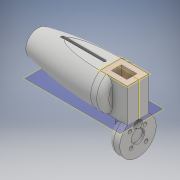
# Autodesk Inventor part: Halterung Motor Neu
Saved by Autodesk Inventor 2019 (Build 230136000, 136)
## iProperties
Created: 2017-06-08
Part Number: Halterung Motor Neu
Material: Allgemein
Document SubType Name: Modeling
Designer: eule-3
Density: 1 g/cm^3
Appearance: Vorgabe
Author: eule-3
Autodesk Inventor part; units mm, degrees
ref_plane "YZ Plane" through (0, 0, 0) normal (1, 0, 0) x (0, 1, 0)
ref_plane "XZ Plane" through (0, 0, 0) normal (0, 1, 0) x (-1, 0, 0)
ref_plane "XY Plane" through (0, 0, 0) normal (0, 0, 1) x (1, 0, 0)
sketch "Skizze1" plane through (0, 0, 0) normal (0, 0, 1) x (1, 0, 0)
  point P0 (0, 0)
sketch "Skizze2" plane through (0, 0, 0) normal (0, 0, 1) x (1, 0, 0)
  line L0 (0, 0) -> (22.5, 0)
  line L1 (22.5, 0) -> (22.5, 17.5)
  line L2 (22.5, 17.5) -> (0, 17.5)
  line L3 (0, 17.5) -> (0, 0)
  dimension "d0" = 17.5
  dimension "d1" = 22.5
  constraints: 8 end point, 2 parallel, 1 horizontal, 1 perpendicular
  measures "d0" distance of L0.end L1.end
  measures "d1" distance of L1.end L2.end
extrude "Extrusion1" add sketch "Skizze2" along normal blind 28
sketch "Skizze3" plane through (0, 17.5, 0) normal (0, 1, 0) x (1, 0, 0)
  point P0 (0, 0)
sketch "Skizze4" plane through (22.5, 0, 0) normal (1, 0, 0) x (0, 0, -1)
  circle A0 centre (12.1835, 8.75) radius 15
  line L0 (0, 17.5) -> (-28, 17.5) projected
  line L1 (0, 0) -> (-28, 0) projected
  dimension "d4" = 30
  dimension "d5" = 8.75
  dimension "d6" = 8.75
  dimension "d7" = 15
  constraints: 1 centre point
  measures "d4" diameter of A0
  measures "d5" distance from line of A0.centre L0
  measures "d6" distance from line of A0.centre L1
  measures "d7" distance of A0.centre L0.start
extrude "Extrusion2" cut sketch "Skizze4" against normal blind 22.5
sketch "Skizze5" plane through (22.5, 0, 28) normal (1, 0, 0) x (0, 0, -1)
  circle A0 centre (40.1835, 8.75) radius 15
  line L0 (28, 17.5) -> (0, 17.5) projected
  point P0 (28, 0)
  dimension "d10" = 30
  dimension "d11" = 8.75
  dimension "d12" = 15
  constraints: 1 centre point
  measures "d10" diameter of A0
  measures "d11" distance from line of L0 A0.centre
  measures "d12" distance of L0.start A0.centre
extrude "Extrusion3" add sketch "Skizze5" against normal blind 22.5
sketch "Skizze6" plane through (22.5, 0, 28) normal (1, 0, 0) x (0, 0, -1)
  point P0 (28, 0)
sketch "Skizze7" plane through (0, 0, 28) normal (-1, 0, 0) x (0, 0, 1)
  circle A0 centre (-40.1835, 8.75) radius 15
  line L0 (-28, 0) -> (0, 0) projected
  dimension "d15" = 30
  dimension "d16" = 8.75
  dimension "d17" = 15
  constraints: 1 centre point
  measures "d15" diameter of A0
  measures "d16" distance from line of L0 A0.centre
  measures "d17" distance of A0.centre L0.start
extrude "Extrusion4" cut sketch "Skizze7" against normal blind 12.5
sketch "Skizze8" plane through (0, 0, 28) normal (-1, 0, 0) x (0, 0, 1)
  line L0 (-28, 17.4854) -> (-24, 17.4854)
  line L1 (-24, 17.4854) -> (-24, 0)
  line L2 (-24, 0) -> (-28, 0)
  line L3 (-28, 0) -> (-28, 17.4854)
  constraints: 8 end point, 2 parallel, 1 horizontal, 1 perpendicular
extrude "Extrusion5" add sketch "Skizze8" against normal blind 12.5
sketch "Skizze9" plane through (12.5, 0, 28) normal (-1, 0, 0) x (0, 0, 1)
  point P0 (-28, 0)
sketch "Skizze10" plane through (12.5, 0, 28) normal (-1, 0, 0) x (0, 0, 1)
  line L0 (-28, 17.5) -> (0, 17.5) projected
  arc A0 (-28, 17.5) -> (-28, 0) centre (-40.1835, 8.75) ccw projected
  line L1 (-28, 0) -> (-28, 17.4854) projected
  line L2 (-40.1835, 8.75) -> (-28, 8.7427)
  line L3 (-40.1835, 23.75) -> (-40.1835, 8.75)
  line L4 (-55.1835, 8.75) -> (-40.1835, 8.75)
  line L5 (-40.1835, 8.75) -> (-40.1835, -6.25)
  point P0 (-34.5249, 14.4052)
  point P1 (-33.468, 2.0305)
  point P2 (-46.901, 15.4675)
  point P3 (-45.8403, 3.0931)
  dimension "d38" = 9.5
  constraints: 8 end point, 3 point on circle, 1 horizontal, 1 midpoint, 1 perpendicular, 1 point on line, 1 vertical
  measures "d38" distance of L2.start point (-46.901, 15.468)
hole "Bohrung1" at (12.5, 15.4675, -18.901) at (12.5, 2.0305, -5.468) at (12.5, 3.0931, -17.8403) at (12.5, 14.4052, -6.5249) direction (1, 0, 0) diameter 3 end through all
sketch "Skizze11" plane through (12.5, 0, 28) normal (-1, 0, 0) x (0, 0, 1)
  point P0 (-28, 0)
sketch "Skizze12" plane through (0, 0, 28) normal (0, 0, 1) x (1, 0, 0)
  line L0 (4.8, 12.85) -> (17.5, 12.85)
  line L1 (17.5, 12.85) -> (17.5, 4.65)
  line L2 (17.5, 4.65) -> (4.8, 4.65)
  line L3 (4.8, 4.65) -> (4.8, 12.85)
  line L4 (22.5, 17.5) -> (0, 17.5) projected
  line L5 (22.5, 0) -> (22.5, 17.5) projected
  line L6 (0, 17.5) -> (0, 0) projected
  line L7 (0, 0) -> (22.5, 0) projected
  dimension "d78" = 4.65
  dimension "d79" = 4.65
  dimension "d111" = 5
  dimension "d112" = 12.7
  constraints: 8 end point, 2 parallel, 1 horizontal, 1 perpendicular
  measures "d78" distance between parallel lines of L4 L0
  measures "d79" distance between parallel lines of L7 L2
  measures "d111" distance between parallel lines of L5 L1
  measures "d112" distance of L1.end L2.end
extrude "Extrusion6" cut sketch "Skizze12" against normal blind 30 contours L0 L1 L2 L3
sketch "Skizze13" plane through (12.5, 0, 28) normal (-1, 0, 0) x (0, 0, 1)
  circle A0 centre (-31.75, 8.75) radius 2.25
  line L0 (-30, 12.85) -> (-30, 4.65) projected
  point P0 (-28, 0)
  dimension "d71" = 1.75
  constraints: 1 centre point, 1 coincident
  measures "d71" distance from line of L0 A0.centre
extrude "Extrusion7" cut sketch "Skizze13" against normal blind 10
sketch "Skizze14" plane through (22.5, 0, 28) normal (1, 0, 0) x (0, 0, -1)
  line L0 (28, 17.5) -> (0, 17.5) projected
  circle A0 centre (31.75, 8.75) radius 2.25 projected
  arc A1 (28, 0) -> (28, 17.5) centre (40.1835, 8.75) ccw projected
  circle A2 centre (40.1835, 8.75) radius 5
  dimension "d57" = 10
  constraints: 1 centre point, 1 coincident
  measures "d57" diameter of A2
extrude "Extrusion8" cut sketch "Skizze14" against normal blind 1.5 contours A2
chamfer "Fase1" distance 0.5 angle 45 1 edges at (22.5, 8.75, -7.1835)
chamfer "Fase2" distance 0.5 angle 45 4 edges at (12.5, 15.4675, -20.401) (12.5, 14.4052, -8.0249) (12.5, 2.0305, -6.968) (12.5, 3.0931, -19.3403)
sketch "Skizze16" plane through (12.5, 0, 28) normal (-1, 0, 0) x (0, 0, 1)
  circle A0 centre (-31.75, 8.75) radius 2.25 projected
  line L0 (-30, 4.65) -> (-30, 7.3358) projected
  line L1 (-31.75, 10.825) -> (-30, 10.825)
  line L2 (-30, 10.825) -> (-30, 5.9929)
  line L3 (-30, 5.9929) -> (-31.75, 5.9929)
  line L4 (-31.75, 5.9929) -> (-31.75, 10.825)
  point P0 (-28, 0)
  point P1 (-31.75, 6.5)
  constraints: 8 end point, 2 parallel, 1 coincident, 1 horizontal, 1 midpoint, 1 perpendicular, 1 other
extrude "Extrusion9" cut sketch "Skizze16" against normal blind 5 contours L0 L3 L4 A0 | A0 L4 L1 L2 | A0 L1 L2
sketch "Skizze17" plane through (0, 0, 28) normal (0, 0, 1) x (1, 0, 0)
  point P0 (0, 0)
sketch "Skizze18" plane through (0, 0, -2) normal (0, 0, 1) x (1, 0, 0)
  line L0 (12.5, 6.5) -> (17.5, 6.5) projected
  line L1 (12.5, 5.9929) -> (17.5, 5.9929) projected
  line L2 (12.5, 6.5) -> (17.5, 6.5)
  line L3 (17.5, 6.5) -> (17.5, 5.9929)
  line L4 (17.5, 5.9929) -> (12.5, 5.9929)
  line L5 (12.5, 5.9929) -> (12.5, 6.5)
  point P0 (0, 0)
  constraints: 8 end point, 2 parallel, 1 horizontal, 1 perpendicular
extrude "Extrusion10" add sketch "Skizze18" against normal blind 5
sketch "Skizze19" plane through (22.5, 0, 28) normal (1, 0, 0) x (0, 0, -1)
  circle A0 centre (31.7095, 8.8101) radius 3.5
  point P0 (28, 0)
  dimension "d80" = 7
  constraints: 1 centre point
  measures "d80" diameter of A0
extrude "Extrusion11" cut sketch "Skizze19" against normal blind 5
sketch "Skizze20" plane through (0, 0, 28) normal (0, 0, 1) x (1, 0, 0)
  line L0 (17.5, 4.65) -> (4.8, 4.65) projected
  line L1 (4.8, 12.85) -> (17.5, 12.85) projected
  line L2 (4.8, 4.65) -> (4.8, 12.85) projected
  line L3 (17.5, 12.85) -> (17.5, 4.65) projected
  point P0 (0, 0)
sketch "Skizze21" plane through (0, 0, 28) normal (-1, 0, 0) x (0, 0, 1)
  line L0 (-28, 0) -> (-28, 17.4854) projected
  line L1 (-28, 17.5) -> (0, 17.5) projected
  line L2 (-28, 0) -> (0, 0)
  line L3 (0, 0) -> (0, 17.5)
  line L4 (0, 17.5) -> (-28, 17.5)
  line L5 (-28, 17.5) -> (-28, 0)
  arc A0 (0, 17.5) -> (-28, 17.5) centre (-14, 8.75) ccw
  arc A1 (-28, 0) -> (0, 0) centre (-14, 8.75) ccw
  point P0 (-28.6212, 17.5)
  dimension "d85" = 28
  dimension "d86" = 17.5
  dimension "d87" = 16.5095
  constraints: 8 end point, 4 point on circle, 2 centre point, 2 coincident, 2 parallel, 1 horizontal, 1 perpendicular
  measures "d85" distance between parallel lines of L3 L0
  measures "d86" distance between parallel lines of L2 L1
  measures "d87" radius of A0
extrude "Extrusion12" add sketch "Skizze21" against normal blind 10 contours L2 A1 | A0 L1
fillet "Rundung1" radius 5 2 edges at (10, -7.7595, 14) (10, 25.2595, 14)
sketch "Skizze22" plane through (0, 0, 28) normal (0, 0, 1) x (1, 0, 0)
  point P0 (0, 0)
ref_plane "Arbeitsebene1" through (13, 8.75, 0) normal (0, -1, 0) x (1, 0, 0)
sketch "Skizze23" plane through (13, 8.75, 0) normal (0, -1, 0) x (1, 0, 0)
  line L0 (-13, 28) -> (-13, 0) projected
  line L1 (-73, 14) -> (-73, 24)
  line L2 (-13, 14) -> (-13, 30.5095)
  line L3 (-13, 0) -> (-8, 0) projected
  arc A0 (-13, 30.5095) -> (-73, 24) centre (-13, -249.2642) ccw
  line L4 (-73, 14) -> (-13, 14)
  dimension "d92" = 60
  dimension "d93" = 10
  dimension "d94" = 16.5095
  dimension "d95" = 14
  constraints: 6 end point, 2 point on circle, 2 vertical, 1 centre point, 1 line through centre, 1 midpoint
  measures "d92" distance of L2.start L1.start
  measures "d93" distance of L1.start L1.end
  measures "d94" distance of L2.start L2.end
  measures "d95" distance from line of L3 L1.start
revolve "Umdrehung1" add sketch "Skizze23" angle 360 about axis through (-60, 8.75, 14) along (1, 0, 0) separate body
sketch "Skizze25" plane through (0, 8.75, 14) normal (1, 0, 0) x (0, 0, -1)
  point P0 (14, -8.75)
ref_plane "Arbeitsebene2" through (0, 0, 28) normal (0, 0, 1) x (1, 0, 0)
ref_plane "Arbeitsebene3" through (6.25, 17.4854, 0) normal (0, 0, -1) x (-1, 0, 0)
split "Trennen3" plane through (6.25, 17.4854, 0) removes the side toward (0, 0, -1) bodies 2
split "Trennen4" plane through (0, 0, 28) removes the side toward (0, 0, 1) bodies 2
sketch "Skizze27" plane through (-60, 8.75, 14) normal (-1, 0, 0) x (0, 0, 1)
  line L0 (14, 4.1) -> (-14, 4.1) projected
  line L1 (-14, -8.7501) -> (-14, 8.7501) projected
  point P0 (-14, -8.75)
  point P1 (0, 0)
  point P2 (0, 4.1)
  point P3 (-14, 0)
  constraints: 2 midpoint, 1 horizontal alignment, 1 vertical alignment
hole "Bohrung2" at (-60, 8.75, 14) direction (1, 0, 0) diameter 11 depth 50 tip angle 118 counterbore diameter 13 counterbore depth 8 bodies 2
sketch "Skizze28" plane through (0, -0.0001, 0) normal (0, 0, -1) x (-1, 0, 0)
  line L0 (5, 8.7501) -> (40, 8.7501) construction
  line L1 (5, 7.7501) -> (40, 7.7501)
  line L2 (40, 9.7501) -> (5, 9.7501)
  arc A0 (5, 9.7501) -> (5, 7.7501) centre (5, 8.7501) ccw
  arc A1 (40, 7.7501) -> (40, 9.7501) centre (40, 8.7501) ccw
  line L3 (76.5004, 8.7501) -> (-39.0025, 8.7501) projected
  line L4 (0, 0) -> (0, 17.5001) projected
  point P0 (0, 0.0001)
  point P1 (22.5, 8.7501)
  dimension "d106" = 35
  dimension "d107" = 1
  dimension "d108" = 5
  constraints: 8 end point, 4 point on circle, 4 tangent, 2 centre point, 1 collinear, 1 horizontal, 1 midpoint, 1 parallel
  measures "d106" distance of L2.start L2.end
  measures "d107" radius of A0
  measures "d108" distance from line of L4 L0.start
extrude "Extrusion13" cut sketch "Skizze28" against normal through all bodies 2
fillet "Rundung2" radius 5 1 edges at (12.5, 8.75, -27.1835)
